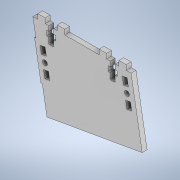
# Autodesk Inventor part: tc_support_front
Saved by Autodesk Inventor 2020.1 (Build 241239000, 239)
## iProperties
Created: 2019-07-16
Part Number: tc_support_front
Material: Acier inoxydable
Document SubType Name: Modeling
Designer: Thibault
Density: 8 g/cm^3
Appearance: Semi-poli
anchor_dist_b: 36.000 mm
anchor_dist_a: 2,000 mm
anchor_dist_top_a: 8.000 mm
tilt_angle: 10.00 deg
Author: Thibault
Autodesk Inventor part; units mm, degrees
ref_plane "YZ Plane" through (0, 0, 0) normal (1, 0, 0) x (0, 1, 0)
ref_plane "XZ Plane" through (0, 0, 0) normal (0, 1, 0) x (-1, 0, 0)
ref_plane "XY Plane" through (0, 0, 0) normal (0, 0, 1) x (1, 0, 0)
sketch "Anchor (screw side)" plane through (0, 0, 0) normal (0, 0, 1) x (1, 0, 0)
  circle A0 centre (93.7814, 50.2592) radius 1
  line L0 (91.2814, 51.2592) -> (88.2814, 51.2592)
  line L1 (88.2814, 51.2592) -> (88.2814, 49.2592)
  line L2 (88.2814, 49.2592) -> (91.2814, 49.2592)
  line L3 (91.2814, 49.2592) -> (91.2814, 51.2592)
  line L4 (99.2814, 51.2592) -> (96.2814, 51.2592)
  line L5 (96.2814, 51.2592) -> (96.2814, 49.2592)
  line L6 (96.2814, 49.2592) -> (99.2814, 49.2592)
  line L7 (99.2814, 49.2592) -> (99.2814, 51.2592)
  line L8 (91.2814, 51.2592) -> (96.2814, 49.2592) construction
  line L9 (96.2814, 51.2592) -> (91.2814, 49.2592) construction
  line L10 (86.2814, 53.2592) -> (101.2814, 53.2592) construction
  line L11 (101.2814, 53.2592) -> (101.2814, 47.2592) construction
  line L12 (101.2814, 47.2592) -> (86.2814, 47.2592) construction
  line L13 (86.2814, 47.2592) -> (86.2814, 53.2592) construction
  point P0 (103.5798, 50.1132)
  dimension "d27" = 2
  dimension "d28" = 3
  dimension "d29" = 2
  dimension "d30" = 3
  dimension "d32" = 5
  dimension "d34" = 2
  dimension "d35_1" = 2
  dimension "d36_1" = 2
  dimension "d37" = 2
  measures "d27" diameter of A0
  measures "d28" distance of L2.end L1.end
  measures "d29" distance of L1.end L0.end
  measures "d30" distance of L6.end L5.end
  measures "d32" distance between parallel lines of L5 L3
  measures "d34" distance between parallel lines of L0 L10
  measures "d35_1" distance between parallel lines of L12 L2
  measures "d36_1" distance between parallel lines of L11 L7
  measures "d37" distance between parallel lines of L13 L1
sketch "Anchor (nut side)" plane through (0, 0, 0) normal (0, 0, 1) x (1, 0, 0)
  line L0 (10, 0) -> (8.5, 0)
  line L1 (8.5, 0) -> (8.5, -2)
  line L2 (8.5, -2) -> (9.3, -2)
  line L3 (9.3, -2) -> (9.3, -4)
  line L4 (5.7, -4) -> (5.7, -2)
  line L5 (5.7, -2) -> (6.5, -2)
  line L6 (6.5, -2) -> (6.5, 0)
  line L7 (6.5, 0) -> (5, 0)
  line L8 (2, 0) -> (2, 2)
  line L9 (2, 0) -> (3, 0) construction
  line L10 (2, 2) -> (5, 2)
  line L11 (5, 2) -> (5, 0)
  line L12 (5, 2) -> (7, 2) construction
  line L13 (10, 0) -> (10, 2)
  line L14 (10, 2) -> (13, 2)
  line L15 (13, 2) -> (13, 0)
  line L16 (0, 0) -> (2, 0)
  line L17 (13, 0) -> (15, 0)
  line L18 (5.7, -4) -> (6.5, -4)
  line L19 (9.3, -4) -> (8.5, -4)
  line L20 (6.5, -4) -> (6.5, -6.25)
  line L21 (8.5, -4) -> (8.5, -6.25)
  line L22 (6.75, -6.5) -> (7.5, -6.5)
  arc A0 (6.5, -6.25) -> (6.75, -6.5) centre (6.75, -6.25) ccw
  arc A1 (8.25, -6.5) -> (8.5, -6.25) centre (8.25, -6.25) ccw
  line L23 (7.5, -7.2938) -> (7.5, -4.9797)
  line L24 (7.5, -6.5) -> (8.25, -6.5)
  point P0 (9.1321, -0.6227)
  point P1 (6.5, -6.5)
  point P2 (8.5, -6.5)
  dimension "d3" = 2
  dimension "d7" = 5
  dimension "d10" = 1.5
  dimension "d11" = 2
  dimension "d12" = 0.8
  dimension "d13" = 2
  dimension "d14" = 0.8
  dimension "d15" = 2
  dimension "d18" = 2
  dimension "d19" = 0.8
  dimension "d20" = 0.8
  dimension "d21" = 2.5
  dimension "d22" = 2.5
  dimension "d23" = 2
  dimension "d38" = 2
  dimension "d39" = 0.25
  dimension "d118" = 2
  dimension "d120" = 3
  measures "d3" distance of L16.start L8.start
  measures "d7" distance of L7.end L0.start
  measures "d10" distance of L0.start L0.end
  measures "d11" distance of L0.end L1.end
  measures "d12" distance of L1.end L2.end
  measures "d13" distance of L2.end L3.end
  measures "d14" distance of L4.end L5.end
  measures "d15" distance of L6.end L0.end
  measures "d18" distance of L15.end L17.end
  measures "d19" distance of L4.start L18.end
  measures "d20" distance of L3.end L19.end
  measures "d21" distance of L18.end point (6.5, -6.5)
  measures "d22" distance of L19.end point (8.5, -6.5)
  measures "d23" distance of L18.end L19.end
  measures "d38" distance between parallel lines of L16 L10
  measures "d39" radius of A0
  measures "d118" distance between parallel lines of L0 L14
  measures "d120" distance of L8.end L10.end
derived "shared_parameters.ipt"
sketch "Esquisse1" plane through (0, 0, 0) normal (0, 0, 1) x (1, 0, 0)
  line L0 (83.0158, -42.9578) -> (78.4658, -17.1534)
  line L1 (83.0158, -42.9578) -> (44.1735, -49.8067)
  line L2 (-2.0657, -1.8526) -> (7.9343, -1.7975) construction
  line L3 (39.6399, -24.0953) -> (38.4158, -17.1534)
  line L4 (53.4158, -17.1534) -> (63.4658, -17.1534)
  line L5 (39.0899, -24.1923) -> (41.6946, -38.9644)
  line L6 (39.0899, -24.1923) -> (39.6399, -24.0953)
  line L7 (44.1735, -49.8067) -> (42.2446, -38.8674)
  line L8 (41.6946, -38.9644) -> (42.2446, -38.8674)
  circle A0 centre (76.8302, -25.1534) radius 1
  line L9 (76.2795, -27.789) -> (76.8004, -30.7435)
  line L10 (76.8004, -30.7435) -> (78.77, -30.3962)
  line L11 (78.77, -30.3962) -> (78.2491, -27.4418)
  line L12 (78.2491, -27.4418) -> (76.2795, -27.789)
  line L13 (74.8903, -19.9106) -> (75.4112, -22.865)
  line L14 (75.4112, -22.865) -> (77.3808, -22.5177)
  line L15 (77.3808, -22.5177) -> (76.8599, -19.5633)
  line L16 (76.8599, -19.5633) -> (74.8903, -19.9106)
  line L17 (76.2795, -27.789) -> (77.3808, -22.5177) construction
  line L18 (75.4112, -22.865) -> (78.2491, -27.4418) construction
  line L19 (75.1781, -33.0604) -> (72.5734, -18.2883) construction
  line L20 (72.5734, -18.2883) -> (78.4822, -17.2464) construction
  line L21 (78.4822, -17.2464) -> (81.0869, -32.0185) construction
  line L22 (81.0869, -32.0185) -> (75.1781, -33.0604) construction
  circle A1 centre (43.3467, -31.0574) radius 1
  line L23 (43.8974, -28.4218) -> (43.3764, -25.4673)
  line L24 (43.3764, -25.4673) -> (41.4068, -25.8146)
  line L25 (41.4068, -25.8146) -> (41.9278, -28.769)
  line L26 (41.9278, -28.769) -> (43.8974, -28.4218)
  line L27 (45.2866, -36.3002) -> (44.7656, -33.3458)
  line L28 (44.7656, -33.3458) -> (42.796, -33.6931)
  line L29 (42.796, -33.6931) -> (43.3169, -36.6475)
  line L30 (43.3169, -36.6475) -> (45.2866, -36.3002)
  line L31 (43.8974, -28.4218) -> (42.796, -33.6931) construction
  line L32 (44.7656, -33.3458) -> (41.9278, -28.769) construction
  line L33 (44.9987, -23.1504) -> (47.6035, -37.9225) construction
  line L34 (47.6035, -37.9225) -> (41.6946, -38.9644) construction
  line L35 (41.6946, -38.9644) -> (39.0899, -24.1923) construction
  line L36 (39.0899, -24.1923) -> (44.9987, -23.1504) construction
  line L37 (48.4158, -17.1534) -> (46.9158, -17.1534)
  line L38 (46.9158, -17.1534) -> (46.9158, -19.1534)
  line L39 (46.9158, -19.1534) -> (47.7158, -19.1534)
  line L40 (47.7158, -19.1534) -> (47.7158, -21.1534)
  line L41 (44.1158, -21.1534) -> (44.1158, -19.1534)
  line L42 (44.1158, -19.1534) -> (44.9158, -19.1534)
  line L43 (44.9158, -19.1534) -> (44.9158, -17.1534)
  line L44 (44.9158, -17.1534) -> (43.4158, -17.1534)
  line L45 (40.4158, -17.1534) -> (40.4158, -15.1534)
  line L46 (40.4158, -17.1534) -> (41.4158, -17.1534) construction
  line L47 (40.4158, -15.1534) -> (43.4158, -15.1534)
  line L48 (43.4158, -15.1534) -> (43.4158, -17.1534)
  line L49 (43.4158, -15.1534) -> (45.4158, -15.1534) construction
  line L50 (48.4158, -17.1534) -> (48.4158, -15.1534)
  line L51 (48.4158, -15.1534) -> (51.4158, -15.1534)
  line L52 (51.4158, -15.1534) -> (51.4158, -17.1534)
  line L53 (38.4158, -17.1534) -> (40.4158, -17.1534)
  line L54 (51.4158, -17.1534) -> (53.4158, -17.1534)
  line L55 (44.1158, -21.1534) -> (44.9158, -21.1534)
  line L56 (47.7158, -21.1534) -> (46.9158, -21.1534)
  line L57 (44.9158, -21.1534) -> (44.9158, -23.4034)
  line L58 (46.9158, -21.1534) -> (46.9158, -23.4034)
  line L59 (45.1658, -23.6534) -> (45.9158, -23.6534)
  arc A2 (44.9158, -23.4034) -> (45.1658, -23.6534) centre (45.1658, -23.4034) ccw
  arc A3 (46.6658, -23.6534) -> (46.9158, -23.4034) centre (46.6658, -23.4034) ccw
  line L60 (45.9158, -24.4472) -> (45.9158, -22.1331)
  line L61 (45.9158, -23.6534) -> (46.6658, -23.6534)
  line L62 (73.4658, -17.1534) -> (71.9658, -17.1534)
  line L63 (71.9658, -17.1534) -> (71.9658, -19.1534)
  line L64 (71.9658, -19.1534) -> (72.7658, -19.1534)
  line L65 (72.7658, -19.1534) -> (72.7658, -21.1534)
  line L66 (69.1658, -21.1534) -> (69.1658, -19.1534)
  line L67 (69.1658, -19.1534) -> (69.9658, -19.1534)
  line L68 (69.9658, -19.1534) -> (69.9658, -17.1534)
  line L69 (69.9658, -17.1534) -> (68.4658, -17.1534)
  line L70 (65.4658, -17.1534) -> (65.4658, -15.1534)
  line L71 (65.4658, -17.1534) -> (66.4658, -17.1534) construction
  line L72 (65.4658, -15.1534) -> (68.4658, -15.1534)
  line L73 (68.4658, -15.1534) -> (68.4658, -17.1534)
  line L74 (68.4658, -15.1534) -> (70.4658, -15.1534) construction
  line L75 (73.4658, -17.1534) -> (73.4658, -15.1534)
  line L76 (73.4658, -15.1534) -> (76.4658, -15.1534)
  line L77 (76.4658, -15.1534) -> (76.4658, -17.1534)
  line L78 (63.4658, -17.1534) -> (65.4658, -17.1534)
  line L79 (76.4658, -17.1534) -> (78.4658, -17.1534)
  line L80 (69.1658, -21.1534) -> (69.9658, -21.1534)
  line L81 (72.7658, -21.1534) -> (71.9658, -21.1534)
  line L82 (69.9658, -21.1534) -> (69.9658, -23.4034)
  line L83 (71.9658, -21.1534) -> (71.9658, -23.4034)
  line L84 (70.2158, -23.6534) -> (70.9658, -23.6534)
  arc A4 (69.9658, -23.4034) -> (70.2158, -23.6534) centre (70.2158, -23.4034) ccw
  arc A5 (71.7158, -23.6534) -> (71.9658, -23.4034) centre (71.7158, -23.4034) ccw
  line L85 (70.9658, -24.4472) -> (70.9658, -22.1331)
  line L86 (70.9658, -23.6534) -> (71.7158, -23.6534)
  point P0 (76.8302, -25.1534)
  point P1 (43.3467, -31.0574)
  point P2 (78.4658, -17.1534)
  dimension "d44" = 13.1081
  dimension "d45" = 1.4416
  dimension "d55" = 40.05
  constraints: 18 end point, 3 horizontal, 2 perpendicular, 2 point on line, 1 collinear, 1 parallel, 14 other
  measures "d55" distance of L3.end L0.end
extrude "Extrusion1" add sketch "Esquisse1" along normal blind 2
equation "\"d44\" = extra_height_back"
equation "\"d55\" = tc_base_back_width"
equation "\"d35\" = sheet_thickness"
equation "\"extra_height_back\" = 13.108056"
equation "\"tc_base_back_width\" = 40.05"
equation "\"sheet_thickness\" = 2"
